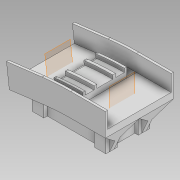
# Autodesk Inventor part: Slope_HighEnd
Saved by Autodesk Inventor 2021 (Build 250183000, 183)
## iProperties
Created: 2021-03-11
Part Number: Slope_HighEnd
Material: 一般
Document SubType Name: Modeling
Designer: kumagai
Density: 1 g/cm^3
Appearance: 既定
Author: kumagai
Autodesk Inventor part; units mm, degrees
ref_plane "YZ Plane" through (0, 0, 0) normal (1, 0, 0) x (0, 1, 0)
ref_plane "XY Plane" through (0, 0, 0) normal (0, 0, 1) x (1, 0, 0)
derived "SlopeProfile.ipt"
sketch "スケッチ1" plane through (0, 0, 0) normal (0, 0, 1) x (1, 0, 0)
  line L0 (0, 14) -> (0, -14)
  line L1 (-14, 0) -> (14, 0)
  line L2 (-268.75, 0) -> (268.75, 0)
  line L3 (-268.75, 0) -> (268.75, 66)
  line L4 (268.75, 66) -> (268.75, 0)
  line L5 (-31.5879, 61.457) -> (-25.6465, 13.0705)
  line L6 (-134.375, 50.6657) -> (-134.375, 8.5939)
  line L7 (23.2129, 72.7486) -> (28.7067, 28.0077)
  line L8 (-244.2356, 29.1492) -> (-240.1953, -3.7549)
  line L9 (134.375, 89.7324) -> (134.375, 45.3233)
  line L10 (239.1121, 78.5758) -> (241.9591, 55.3901)
  line L11 (-27.6764, 5.7379) -> (-27.6764, -11.9933)
  line L12 (27.6764, 6.5088) -> (27.6764, -13.0212)
  line L13 (-268.75, 0) -> (-295.625, 0)
  line L14 (268.75, 66) -> (295.625, 66)
  line L15 (241.0736, 6.6999) -> (241.0736, -9.2827)
  line L16 (-241.0736, -7.7427) -> (-241.0736, -14.414)
  arc A0 (-280.625, 0) -> (-256.9635, 1.4473) centre (-280.625, 194.1449) ccw
  line L17 (-256.3082, 4.3915) -> (-255.7778, 0.0713)
  line L18 (-280.625, 8.6126) -> (-280.625, -11.6883)
  line L19 (-295.625, 14.7784) -> (-295.625, -11.568)
  line L20 (255.3892, 69.0933) -> (256.9398, 56.465)
  line L21 (280.625, 71.1514) -> (280.625, 58.4982)
  line L22 (295.625, 71.9522) -> (295.625, 60.0478)
  arc A1 (280.625, 66) -> (256.9635, 64.5527) centre (280.625, -128.1449) ccw
  line L23 (-13.2739, 35.3851) -> (-12.039, 25.3288)
  line L24 (-43.1495, 32.5373) -> (-41.4451, 18.6566)
  line L25 (12.2235, 39.1691) -> (13.7539, 26.7059)
  line L26 (41.8424, 44.108) -> (43.6336, 29.5201)
  point P0 (0, 0)
  point P1 (-241.0736, 3.3984)
  point P2 (-27.6764, 29.6016)
  point P3 (27.6764, 36.3984)
  point P4 (241.0736, 62.6016)
  point P5 (134.375, 49.5)
  point P6 (-134.375, 16.5)
ref_plane "作業平面1" through (241.0736, 62.6016, 0) normal (0.9925454, 0.1218753, 0) x (-0.1218753, 0.9925454, 0)
sketch "スケッチ2" plane through (241.0736, 62.6016, 0) normal (0.9925454, 0.1218753, 0) x (-0.1218753, 0.9925454, 0)
  line L0 (16.0942, 0) -> (-7.2657, 0) projected
  line L1 (3.2, 19) -> (-5.2, 19)
  line L2 (-5.2, 19) -> (-5.2, -19)
  line L3 (-5.2, -19) -> (3.2, -19)
  line L4 (3.2, -19) -> (3.2, -17)
  line L5 (3.2, -17) -> (0, -17)
  line L6 (0, -17) -> (0, -9.3)
  line L7 (0, -9.3) -> (3.2, -9.3)
  line L8 (3.2, -9.3) -> (3.2, -6.9)
  line L9 (3.2, -6.9) -> (0, -6.9)
  line L10 (0, -6.9) -> (0, 6.9)
  line L11 (0, 6.9) -> (3.2, 6.9)
  line L12 (3.2, 6.9) -> (3.2, 9.3)
  line L13 (3.2, 9.3) -> (0, 9.3)
  line L14 (0, 9.3) -> (0, 17)
  line L15 (0, 17) -> (3.2, 17)
  line L16 (3.2, 17) -> (3.2, 19)
  line L17 (-5.2, 27.5) -> (-5.2, -27.5)
  line L18 (-5.2, -27.5) -> (9, -27.5)
  line L19 (9, -27.5) -> (9, -29.5)
  line L20 (9, -29.5) -> (-11, -29.5)
  line L21 (-11, -29.5) -> (-11, 29.5)
  line L22 (-11, 29.5) -> (9, 29.5)
  line L23 (9, 29.5) -> (9, 27.5)
  line L24 (9, 27.5) -> (-5.2, 27.5)
  line L25 (-11, -29.5) -> (-22.3278, -16)
  line L26 (-22.3278, -16) -> (-23, -16)
  line L27 (-23, -16) -> (-23, -12)
  line L28 (-23, -12) -> (-21.0692, -12)
  line L29 (-21.0692, -12) -> (-11, 0)
  line L30 (-11, 0) -> (-21.0692, 12)
  line L31 (-21.0692, 12) -> (-23, 12)
  line L32 (-23, 12) -> (-23, 16)
  line L33 (-23, 16) -> (-22.3278, 16)
  line L34 (-22.3278, 16) -> (-11, 29.5)
  point P0 (-32.754, 0)
  point P1 (0, 0)
  point P2 (-5.2, 19)
  point P3 (-5.2, -19)
  dimension "d10" = 134.375
  dimension "d25" = 38
  dimension "d26" = 8.4
  dimension "d27" = 3.2
  dimension "d28" = 18.6
  dimension "d29" = 2.4
  dimension "d30" = 2
  dimension "d31" = 59
  dimension "d32" = 2
  dimension "d33" = 20
  dimension "d34" = 5.8
  dimension "d36" = 5.8
  dimension "d53" = 40
  dimension "d54" = 40
  dimension "d55" = 4
  dimension "d56" = 12
  dimension "d101" = 32
  constraints: 68 end point, 21 perpendicular, 6 point on line, 3 collinear, 3 horizontal, 3 vertical, 2 midpoint, 1 parallel, 11 other
  measures "d25" distance between parallel lines of L3 L1
  measures "d26" distance between parallel lines of L2 L4
  measures "d27" distance between parallel lines of L6 L4
  measures "d28" distance between parallel lines of L7 L13
  measures "d29" distance between parallel lines of L13 L11
  measures "d30" distance between parallel lines of L1 L15
  measures "d31" distance between parallel lines of L22 L20
  measures "d32" distance between parallel lines of L22 L24
  measures "d33" distance between parallel lines of L21 L19
  measures "d34" distance between parallel lines of L4 L19
  measures "d36" distance between parallel lines of L21 L17
  measures "d53" angle of L21 L25
  measures "d54" angle of L21 L29
  measures "d55" distance between parallel lines of L28 L26
  measures "d56" distance between parallel lines of L27 L21
  measures "d101" distance between parallel lines of L33 L26
sketch "スケッチ3" plane through (0, 0, 0) normal (0, 0, 1) x (1, 0, 0)
  arc A0 (280.625, 66) -> (256.9635, 64.5527) centre (280.625, -128.1449) ccw projected
  line L0 (-268.75, 0) -> (268.75, 66) projected
  line L1 (256.9635, 64.5527) -> (226.1855, 60.7735)
  line L2 (239.1121, 78.5758) -> (241.9591, 55.3901) projected
  line L3 (280.625, 66) -> (310.625, 66)
  line L4 (295.625, 71.9522) -> (295.625, 60.0478) projected
  point P0 (0, 0)
  dimension "d10" = 134.375
  dimension "d37" = 15
  dimension "d39" = 15
  constraints: 4 end point, 1 horizontal, 1 point on line
  measures "d37" distance from line of L1.end L2
  measures "d39" distance from line of L3.end L4
sweep "スイープ1" add profiles "スケッチ2" path "スケッチ3" path curves L1 A0 L3
extrude "押し出し1" cut sketch "スケッチ2" along normal blind 15 and the other way blind 15 contours L10 L9 L8 L7 L6 L5 L4 L3 L2 L0 | L0 L2 L1 L16 L15 L14 L13 L12 L11 L10
ref_plane "作業平面2" through (295.625, 66, 0) normal (1, 0, 0) x (0, 1, 0)
sketch "スケッチ4" plane through (295.625, 66, 0) normal (1, 0, 0) x (0, 1, 0)
  line L0 (3.2, 19.5) -> (-5.2, 19.5)
  line L1 (-5.2, 19.5) -> (-5.2, -19.5)
  line L2 (-5.2, -19.5) -> (3.2, -19.5)
  line L3 (3.2, -19.5) -> (3.2, 19.5)
  line L4 (5.9522, 0) -> (-5.9522, 0) projected
  point P0 (-66, 0)
  point P1 (0, 0)
  dimension "d10" = 134.375
  dimension "d46" = 39
  dimension "d47" = 3.2
  dimension "d48" = 8.4
  constraints: 8 end point, 2 parallel, 1 horizontal, 1 perpendicular, 1 other
  measures "d46" distance between parallel lines of L2 L0
  measures "d47" distance from line of point (0, 0) L3
  measures "d48" distance between parallel lines of L1 L3
extrude "押し出し2" cut sketch "スケッチ4" along normal blind 15 and the other way blind 15
ref_plane "作業平面3" through (0, 33, 0) normal (0, 1, 0) x (-1, 0, 0)
sketch "スケッチ7" plane through (0, 33, 0) normal (0, 1, 0) x (-1, 0, 0)
  line L0 (-425.875, 0) -> (415.875, 0) projected
  line L1 (-295.625, -26.6) -> (-295.625, 26.6) projected
  line L2 (-290.625, -19) -> (-300.625, -19)
  line L3 (-300.625, -19) -> (-300.625, -9)
  line L4 (-300.625, -9) -> (-290.625, -9)
  line L5 (-290.625, -9) -> (-290.625, -19)
  line L6 (-236.875, -19) -> (-246.875, -19)
  line L7 (-246.875, -19) -> (-246.875, -9)
  line L8 (-246.875, -9) -> (-236.875, -9)
  line L9 (-236.875, -9) -> (-236.875, -19)
  line L10 (-290.625, 9) -> (-300.625, 9)
  line L11 (-300.625, 9) -> (-300.625, 19)
  line L12 (-300.625, 19) -> (-290.625, 19)
  line L13 (-290.625, 19) -> (-290.625, 9)
  line L14 (-236.875, 9) -> (-246.875, 9)
  line L15 (-246.875, 9) -> (-246.875, 19)
  line L16 (-246.875, 19) -> (-236.875, 19)
  line L17 (-236.875, 19) -> (-236.875, 9)
  line L18 (-231.875, -16) -> (-305.625, -16)
  line L19 (-305.625, -16) -> (-305.625, -12)
  line L20 (-305.625, -12) -> (-231.875, -12)
  line L21 (-231.875, -12) -> (-231.875, -16)
  line L22 (-231.875, 12) -> (-305.625, 12)
  line L23 (-305.625, 12) -> (-305.625, 16)
  line L24 (-305.625, 16) -> (-231.875, 16)
  line L25 (-231.875, 16) -> (-231.875, 12)
  line L26 (-239.875, 9) -> (-243.875, 9)
  line L27 (-243.875, 9) -> (-243.875, -9)
  line L28 (-243.875, -9) -> (-239.875, -9)
  line L29 (-239.875, -9) -> (-239.875, 9)
  line L30 (-293.625, 9) -> (-297.625, 9)
  line L31 (-297.625, 9) -> (-297.625, -9)
  line L32 (-297.625, -9) -> (-293.625, -9)
  line L33 (-293.625, -9) -> (-293.625, 9)
  point P0 (0, 0)
  point P1 (-297.625, 9)
  point P2 (-293.625, -9)
  point P3 (-243.875, 9)
  point P4 (-239.875, -9)
  point P5 (-236.875, -12)
  point P6 (-246.875, -12)
  point P7 (-290.625, -12)
  point P8 (-300.625, -12)
  point P9 (-300.625, -16)
  point P10 (-290.625, -16)
  point P11 (-236.875, 16)
  point P12 (-246.875, 16)
  point P13 (-290.625, 16)
  point P14 (-300.625, 16)
  point P15 (-300.625, 12)
  point P16 (-290.625, 12)
  point P17 (-246.875, 12)
  point P18 (-236.875, 12)
  dimension "d80" = 10
  dimension "d82" = 43.75
  dimension "d87" = 4
  dimension "d88" = 3
  dimension "d89" = 5
  dimension "d90" = 5
  dimension "d95" = 3
  dimension "d96" = 4
  dimension "d97" = 3
  dimension "d98" = 4
  dimension "d104" = 38
  constraints: 64 end point, 10 collinear, 9 point on line, 2 horizontal, 2 parallel, 2 perpendicular, 1 vertical, 5 other
  measures "d80" distance of L2.start L2.end
  measures "d82" distance between parallel lines of L7 L5
  measures "d87" distance between parallel lines of L20 L18
  measures "d88" distance between parallel lines of L20 L8
  measures "d89" distance between parallel lines of L9 L21
  measures "d90" distance between parallel lines of L19 L3
  measures "d95" distance between parallel lines of L17 L29
  measures "d96" distance between parallel lines of L29 L27
  measures "d97" distance between parallel lines of L11 L31
  measures "d98" distance between parallel lines of L31 L33
  measures "d104" distance between parallel lines of L2 L12
extrude "押し出し8" add sketch "スケッチ7" along normal up to next contours L10 L11 L22 L1 | L4 L1 L20 L3 | L4 L5 L20 L1 | L1 L22 L13 L10 | L20 L5 L18 L1 | L1 L18 L3 L20 | L22 L11 L24 L1 | L1 L24 L13 L22 | L22 L23 L24 L11 | L3 L18 L19 L20 | L14 L15 L22 L17 | L8 L9 L20 L7 | L18 L5 L2 L1 | L1 L2 L3 L18 | L20 L7 L18 L5 | L24 L11 L12 L1 | L1 L12 L13 L24 | L13 L24 L15 L22 | L20 L9 L18 L7 | L15 L24 L17 L22 | L20 L21 L18 L9 | L15 L16 L17 L24 | L17 L24 L25 L22
extrude "押し出し9" add sketch "スケッチ7" along normal up to next contours L31 L10 L1 L0 | L0 L1 L4 L31 | L1 L10 L33 L0 | L0 L33 L4 L1 | L27 L14 L29 L0 | L0 L29 L8 L27
sketch "スケッチ9" plane through (0, 0, 0) normal (0, 0, 1) x (1, 0, 0)
  line L0 (231.875, 33) -> (236.875, 33) projected
  line L1 (300.625, 33) -> (305.625, 33) projected
  line L2 (227.5261, 49.8555) -> (236.875, 33)
  line L3 (236.875, 33) -> (227.5261, 33)
  line L4 (227.5261, 33) -> (227.5261, 49.8555)
  line L5 (310.625, 55) -> (300.625, 33)
  line L6 (310.625, 33) -> (310.625, 55)
  line L7 (300.625, 33) -> (310.625, 33)
  point P0 (0, 0)
  constraints: 12 end point, 2 point on line, 2 vertical
extrude "押し出し10" cut sketch "スケッチ9" along normal through all both and the other way through all
equation "\"d25\" = RailWidth"
equation "\"d26\" = RailHeight"
equation "\"d27\" = RailDepth"
equation "\"d28\" = InsideWidth"
equation "\"d29\" = InnerWall"
equation "\"d30\" = OuterWall"
equation "\"d34\" = d36"
equation "\"d42\" = ConnectorLength"
equation "\"d47\" = RailDepth"
equation "\"d48\" = RailHeight"
equation "\"d50\" = ConnectorLength"
equation "\"d104\" = RailWidth"
equation "\"d79\" = 0.5 * ViaductHeight"
equation "\"RailWidth\" = 38"
equation "\"RailHeight\" = 8.4"
equation "\"RailDepth\" = 3.2"
equation "\"InsideWidth\" = 18.6"
equation "\"InnerWall\" = 2.4"
equation "\"OuterWall\" = 2"
equation "\"ConnectorLength\" = 15"
equation "\"ViaductHeight\" = 66"
